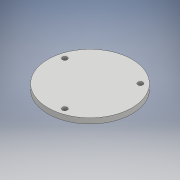
# Autodesk Inventor part: rotate_plate
Saved by Autodesk Inventor 2018 (Build 220112000, 112)
## iProperties
Created: 2019-01-07
Part Number: rotate_plate
Material: 一般
Document SubType Name: Modeling
Designer: lowyu
Density: 1 g/cm^3
Appearance: 既定
Author: lowyu
Autodesk Inventor part; units mm, degrees
ref_plane "YZ Plane" through (0, 0, 0) normal (1, 0, 0) x (0, 1, 0)
ref_plane "XZ Plane" through (0, 0, 0) normal (0, 1, 0) x (-1, 0, 0)
ref_plane "XY Plane" through (0, 0, 0) normal (0, 0, 1) x (1, 0, 0)
sketch "スケッチ1" plane through (0, 0, 0) normal (0, 0, 1) x (1, 0, 0)
  circle A0 centre (-4.0763, -4.0763) radius 35.7
  circle A1 centre (-4.0763, -4.0763) radius 35.7
  circle A2 centre (-33.3097, 3.7568) radius 2.1
  circle A3 centre (3.7568, -33.3097) radius 2.1
  circle A4 centre (17.3241, 17.3241) radius 2.1
  dimension "d0" = 4.2
  dimension "d1" = 4.2
  dimension "d2" = 4.2
  dimension "d3" = 71.4
  constraints: 5 centre point
  measures "d0" diameter of A4
  measures "d1" diameter of A2
  measures "d2" diameter of A3
  measures "d3" diameter of A0
extrude "押し出し1" add sketch "スケッチ1" along normal blind 4.5
sketch "スケッチ3" plane through (-4.0763, -4.0763, 0) normal (0, 0, -1) x (-1, 0, 0)
  circle A0 centre (0, 0) radius 9.75
  circle A1 centre (-5.6569, 5.6569) radius 1.15
  circle A2 centre (-8, 0) radius 1.15
  circle A3 centre (-5.6569, -5.6569) radius 1.15
  circle A4 centre (0, -8) radius 1.15
  circle A5 centre (5.6569, -5.6569) radius 1.15
  circle A6 centre (0, 8) radius 1.15
  circle A7 centre (5.6569, 5.6569) radius 1.15
  circle A8 centre (8, 0) radius 1.15
  circle A9 centre (0, 0) radius 5.5
  point P0 (-4.0763, 4.0763)
  constraints: 10 centre point
extrude "押し出し3" add sketch "スケッチ3" along normal blind 5
